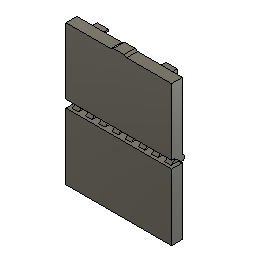
dielectric_frame_box (Autodesk Fusion 360 design; units mm, degrees)
Autodesk Fusion 360 part; units mm, degrees
note: some values were not read from the file. Set by a fixed rule: which face or edge a step refers to.
sketch "Sketch1" plane through (0, 0, 0) normal (0, 0, 1) x (1, 0, 0)
  line L0 (70, 44) -> (-70, 44)
  line L1 (-70, 44) -> (-70, -44)
  line L2 (-70, -44) -> (70, -44)
  line L3 (70, -44) -> (70, 44)
  line L4 (70, 44) -> (-70, -44) construction
  line L5 (-70, 44) -> (70, -44) construction
  dimension "d1" = 140
  dimension "d2" = 88
  constraint horizontal L0
  constraint perpendicular L0 L1
  constraint parallel L0 L2
  constraint parallel L1 L3
  constraint coincident L4 origin
  constraint coincident L5 origin
  measures "d1" distance of L0.start L0.end
  measures "d2" distance of L0.end L1.end
extrude "Extrude1" add sketch "Sketch1" along normal blind 2.5 makes body 1
sketch "Sketch2" plane through (0, 0, 0) normal (0, 0, -1) x (-1, 0, 0)
  line L0 (-70, 44) -> (-70, -44)
  line L1 (-70, -44) -> (70, -44)
  line L2 (70, -44) -> (70, 44)
  line L3 (70, 44) -> (-70, 44)
  line L4 (68.8, 42.8) -> (-68.8, 42.8)
  line L5 (-68.8, 42.8) -> (-68.8, -42.8)
  line L6 (-68.8, -42.8) -> (68.8, -42.8)
  line L7 (68.8, -42.8) -> (68.8, 42.8)
  dimension "d5" = -1.2
sketch "Sketch3" plane through (0, 0, 0) normal (0, 0, -1) x (1, 0, 0)
  line L0 (38, -38.25) -> (38, -31.25)
  line L1 (39, -30.25) -> (42, -30.25)
  line L2 (43, -29.25) -> (43, -26.25)
  line L3 (44, -25.25) -> (51, -25.25)
  line L4 (51, -25.25) -> (51, -38.25)
  line L5 (51, -38.25) -> (38, -38.25)
  line L6 (38, -38.25) -> (38, -40.25)
  line L7 (0, -61) -> (0, 57.3989) construction
  line L8 (91.3753, 0) -> (-120, 0) construction
  arc A0 (42, -30.25) -> (43, -29.25) centre (42, -29.25) ccw
  arc A1 (39, -30.25) -> (38, -31.25) centre (39, -31.25) ccw
  arc A2 (44, -25.25) -> (43, -26.25) centre (44, -26.25) ccw
  line L9 (53, -40.25) -> (53, -25.25)
  line L10 (-68.8, 42.8) -> (-68.8, -42.8)
  line L11 (51, -25.25) -> (53, -25.25)
  line L12 (70, -44) -> (-70, -44) construction
  line L13 (38, -40.25) -> (53, -40.25)
  line L14 (-38, -38.25) -> (-38, -40.25)
  line L15 (-38, -40.25) -> (-53, -40.25)
  line L16 (-53, -40.25) -> (-53, -25.25)
  line L17 (-51, -25.25) -> (-53, -25.25)
  line L18 (-51, -38.25) -> (-38, -38.25)
  line L19 (-51, -25.25) -> (-51, -38.25)
  line L20 (-38, -38.25) -> (-38, -31.25)
  arc A3 (-38, -31.25) -> (-39, -30.25) centre (-39, -31.25) ccw
  line L21 (-39, -30.25) -> (-42, -30.25)
  arc A4 (-43, -29.25) -> (-42, -30.25) centre (-42, -29.25) ccw
  line L22 (-43, -29.25) -> (-43, -26.25)
  arc A5 (-43, -26.25) -> (-44, -25.25) centre (-44, -26.25) ccw
  line L23 (-44, -25.25) -> (-51, -25.25)
  line L24 (38, 38.25) -> (38, 40.25)
  line L25 (38, 40.25) -> (53, 40.25)
  line L26 (51, 25.25) -> (53, 25.25)
  line L27 (53, 40.25) -> (53, 25.25)
  line L28 (51, 38.25) -> (38, 38.25)
  line L29 (51, 25.25) -> (51, 38.25)
  line L30 (38, 38.25) -> (38, 31.25)
  arc A6 (38, 31.25) -> (39, 30.25) centre (39, 31.25) ccw
  line L31 (39, 30.25) -> (42, 30.25)
  arc A7 (43, 29.25) -> (42, 30.25) centre (42, 29.25) ccw
  line L32 (43, 29.25) -> (43, 26.25)
  arc A8 (43, 26.25) -> (44, 25.25) centre (44, 26.25) ccw
  line L33 (44, 25.25) -> (51, 25.25)
  arc A9 (-39, 30.25) -> (-38, 31.25) centre (-39, 31.25) ccw
  line L34 (-39, 30.25) -> (-42, 30.25)
  arc A10 (-42, 30.25) -> (-43, 29.25) centre (-42, 29.25) ccw
  line L35 (-43, 29.25) -> (-43, 26.25)
  arc A11 (-44, 25.25) -> (-43, 26.25) centre (-44, 26.25) ccw
  line L36 (-44, 25.25) -> (-51, 25.25)
  line L37 (-38, 38.25) -> (-38, 31.25)
  line L38 (-51, 38.25) -> (-38, 38.25)
  line L39 (-51, 25.25) -> (-51, 38.25)
  line L40 (-38, 38.25) -> (-38, 40.25)
  line L41 (-38, 40.25) -> (-53, 40.25)
  line L42 (-51, 25.25) -> (-53, 25.25)
  line L43 (-53, 40.25) -> (-53, 25.25)
  point P0 (38, -30.25)
  point P1 (43, -25.25)
  dimension "d10" = 8
  dimension "d11" = 8
  dimension "d12" = 15
  dimension "d13" = 15
  dimension "d14" = 1
  dimension "d15" = 2
  dimension "d48" = 102
  dimension "d49" = 2
  dimension "d85" = 76.5
  constraint vertical L0
  constraint perpendicular L0 L1
  constraint perpendicular L1 L2
  constraint perpendicular L2 L3
  constraint perpendicular L3 L4
  constraint perpendicular L4 L5
  constraint perpendicular L5 L6
  constraint vertical L7
  constraint horizontal L8
  constraint coincident L7 origin
  constraint coincident origin L8
  constraint tangent L1 A0
  constraint tangent L2 A0
  constraint coincident P0 L0
  constraint coincident P0 L1
  constraint tangent L0 A1
  constraint tangent L1 A1
  constraint equal A0 A1
  constraint coincident P1 L2
  constraint coincident P1 L3
  constraint tangent L2 A2
  constraint tangent L3 A2
  constraint equal A0 A2
  constraint equal L4 L5
  constraint perpendicular L4 L11
  constraint perpendicular L9 L13
  constraint symmetric L0.start L7 L14.start
  constraint symmetric L3.end L7 L17.start
  constraint symmetric L4.end L7 L18.start
  constraint symmetric L6.end L7 L14.end
  constraint symmetric L9.start L7 L15.end
  constraint symmetric L7 L1.end L21.end
  constraint symmetric L7 L2.start A4.start
  constraint symmetric L7 A0 A4
  constraint symmetric L7 L0.end L20.end
  constraint symmetric L7 L1.start A3.end
  constraint symmetric L7 A1 A3
  constraint symmetric L7 L2.end L22.end
  constraint symmetric L7 L3.start A5.end
  constraint symmetric L7 A2 A5
  constraint symmetric L7 L9.end L16.end
  constraint symmetric L0.start L8 L24.start
  constraint symmetric L3.end L8 L26.start
  constraint symmetric L4.end L8 L28.start
  constraint symmetric L6.end L8 L24.end
  constraint symmetric L9.start L8 L25.end
  constraint symmetric L8 L1.end L31.end
  constraint symmetric L8 L2.start A7.start
  constraint symmetric L8 A0 A7
  constraint symmetric L8 L0.end L30.end
  constraint symmetric L8 L1.start A6.end
  constraint symmetric L8 A1 A6
  constraint symmetric L8 L2.end L32.end
  constraint symmetric L8 L3.start A8.end
  constraint symmetric L8 A2 A8
  constraint symmetric L8 L9.end L26.end
  constraint symmetric L8 L14.start L37.start
  constraint symmetric L8 L14.end L40.end
  constraint symmetric L8 L15.end L41.end
  constraint symmetric L8 L16.end L42.end
  constraint symmetric L8 L17.start L36.end
  constraint symmetric L8 L18.start L38.start
  constraint symmetric L8 L20.end A9.end
  constraint symmetric L8 A3.end A9.start
  constraint symmetric L8 A3 A9
  constraint symmetric L8 L21.end L34.end
  constraint symmetric L8 A4.start A10.end
  constraint symmetric L8 A4 A10
  constraint symmetric L8 L22.end L35.end
  constraint symmetric L8 A5.end A11.start
  constraint symmetric L8 A5 A11
  measures "d10" distance of L0.start P0
  measures "d11" distance of P1 L3.end
  measures "d12" distance of L6.end L9.start
  measures "d13" distance of L9.start L9.end
  measures "d14" radius of A0
  measures "d15" distance of L0.start L6.end
  measures "d48" distance of L4 L19
  measures "d49" distance of L3.end L9.end
  measures "d85" distance of L5 L28
extrude "Extrude2" add sketch "Sketch3" along normal blind 4 contours L0 L1 L2 L3 L4 L5 A0 A1 A2 | L18 L19 L20 A3 L21 A4 L22 A5 L23 | L28 L29 L30 A6 L31 A7 L32 A8 L33 | A9 L34 A10 L35 A11 L36 L37 L38 L39 bodies 1
extrude "Extrude3" add sketch "Sketch2" along normal blind 12 bodies 1
extrude "Extrude4" add sketch "Sketch3" along normal blind 22 contours L4 L5 L6 L9 L11 L13 | L14 L15 L16 L17 L18 L19 | L24 L25 L26 L27 L28 L29 | L38 L39 L40 L41 L42 L43 bodies 1
ref_plane "WorkPlane1" through (70, 0, -4.75) normal (-1, 0, 0) x (0, -1, 0)
sketch "Sketch4" plane through (70, 0, -10.75) normal (-1, 0, 0) x (0, -1, 0)
  line L0 (44, -1.25) -> (44, 13.25)
  arc A0 (47.2, -3.65) -> (51.2981, 0.6784) centre (49, -1.25) ccw
  circle A1 centre (49, -1.25) radius 1
  line L1 (44, -1.25) -> (47.2, -3.65)
  line L2 (51.2981, 0.6784) -> (44, 9.3759)
  line L3 (44, -1.25) -> (49, -1.25) construction
  dimension "d24" = 3
  dimension "d25" = 2
  dimension "d53" = 5
  dimension "d55" = 140
  constraint concentric A0 A1
  constraint coincident L0.start L1.start
  constraint coincident L0 L2.end
  constraint tangent A0 L2
  constraint tangent A0 L1
  constraint coincident A0.centre A1.centre
  constraint horizontal L3
  measures "d24" radius of A0
  measures "d25" diameter of A1
  measures "d53" horizontal distance of L0.start A0.centre
  measures "d55" angle of L0 L2
extrude "Extrude5" add sketch "Sketch4" along normal mid plane 8.75 separate body makes body 2
pattern_linear "R-Pattern1" count 9 spacing 17.5 along (-1, 0, 0) of bodies 2 makes body 3 at (53.9583, -48.8654, -7.1724) makes body 4 at (36.4583, -48.8654, -7.1724) makes body 5 at (18.9583, -48.8654, -7.1724) makes body 6 at (1.4583, -48.8654, -7.1724) makes body 7 at (-16.0417, -48.8654, -7.1724) makes body 8 at (-33.5417, -48.8654, -7.1724) makes body 9 at (-51.0417, -48.8654, -7.1724) makes body 10 at (-68.5417, -48.8654, -7.1724)
ref_plane "WorkPlane1" through (0, 0, -24) normal (0, 0, -1) x (-1, 0, 0) in component "lid"
sketch "Flat top" plane through (0, 0, -24) normal (0, 0, -1) x (1, 0, 0) in component "lid"
  line L0 (68.8, -42.8) -> (-68.8, -42.8) construction
  line L1 (-68.8, -42.8) -> (-68.8, 42.8) construction
  line L2 (-68.8, 42.8) -> (68.8, 42.8) construction
  line L3 (68.8, 42.8) -> (68.8, -42.8) construction
  line L4 (-70, 44) -> (-70, -44)
  line L5 (-70, -44) -> (70, -44)
  line L6 (70, -44) -> (70, 44)
  line L7 (70, 44) -> (-70, 44)
  line L8 (69.8, -41.8) -> (-69.8, -41.8)
  line L9 (-69.8, -41.8) -> (-69.8, 41.8)
  line L10 (-69.8, 41.8) -> (69.8, 41.8)
  line L11 (69.8, 41.8) -> (69.8, -41.8)
  line L12 (84, 0) -> (65, 0) construction
  constraint horizontal L12
  constraint coincident origin L12
  constraint parallel L0 L8
  constraint parallel L1 L9
  constraint parallel L2 L10
  constraint parallel L3 L11
extrude "Extrude1'" add sketch "Flat top" along normal blind 2.5 separate body contours L4 L5 L6 L7 | L8 L9 L10 L11 makes body 11 in component "lid"
ref_plane "WorkPlane2" through (61.25, -48.5086, -8.6894) normal (1, 0, 0) x (0, 1, 0) in component "lid"
combine "Combine1" operation add target body 1 tool bodies 8 6 3 2 4 5 7 9 10
copy_body "Body->Comp1" bodies 1 removing the originals makes body 12 in component "Component"
ref_plane "WorkPlane3" through (0, 0, -24) normal (0, 0, 1) x (-1, 0, 0) in component "lid"
sketch "Walls" plane through (0, 0, -24) normal (0, 0, 1) x (1, 0, 0) in component "lid"
  line L0 (-68.8, 42.8) -> (-68.8, -42.8)
  line L1 (-68.8, -42.8) -> (68.8, -42.8)
  line L2 (68.8, -42.8) -> (68.8, 42.8)
  line L3 (68.8, 42.8) -> (-68.8, 42.8)
  line L4 (-70, 44) -> (70, 44)
  line L5 (70, 44) -> (70, -44)
  line L6 (70, -44) -> (65.625, -44)
  line L7 (65.625, -44) -> (56.875, -44)
  line L8 (56.875, -44) -> (48.125, -44)
  line L9 (48.125, -44) -> (39.375, -44)
  line L10 (39.375, -44) -> (30.625, -44)
  line L11 (30.625, -44) -> (21.875, -44)
  line L12 (21.875, -44) -> (13.125, -44)
  line L13 (13.125, -44) -> (4.375, -44)
  line L14 (4.375, -44) -> (-4.375, -44)
  line L15 (-4.375, -44) -> (-13.125, -44)
  line L16 (-13.125, -44) -> (-21.875, -44)
  line L17 (-21.875, -44) -> (-30.625, -44)
  line L18 (-30.625, -44) -> (-39.375, -44)
  line L19 (-39.375, -44) -> (-48.125, -44)
  line L20 (-48.125, -44) -> (-56.875, -44)
  line L21 (-56.875, -44) -> (-65.625, -44)
  line L22 (-65.625, -44) -> (-70, -44)
  line L23 (-70, -44) -> (-70, 44)
extrude "Extrude4'" add sketch "Walls" along normal blind 12 separate body makes body 13 in component "lid"
sketch "Hinge profile" plane through (61.25, -46.2271, -22.2758) normal (1, 0, 0) x (0, 0, -1) in component "lid"
  line L0 (1.7242, 2.2271) -> (4.2242, 2.2271)
  circle A0 centre (-10.2758, -2.7729) radius 1.5
  arc A1 (-12.6758, -0.9729) -> (-8.3474, -5.071) centre (-10.2758, -2.7729) ccw
  line L1 (4.2242, 90.2271) -> (4.2242, 2.2271)
  line L2 (1.7242, 2.2271) -> (-10.2758, 2.2271)
  line L3 (-12.6758, -0.9729) -> (-10.2758, 2.2271)
  line L4 (-8.3474, -5.071) -> (0.3502, 2.2271)
  line L5 (-10.2758, -2.7729) -> (-10.2758, 2.2271) construction
  dimension "d59" = 3
  dimension "d60" = 1.5
  dimension "d64" = 5
  dimension "d65" = 12
  dimension "d89" = 140
  constraint coincident A0.centre A1.centre
  constraint coincident L2.end L3.end
  constraint coincident L2 L4.end
  constraint vertical L5
  constraint tangent A1 L4
  constraint tangent A1 L3
  measures "d59" diameter of A0
  measures "d60" distance of A0 A1
  measures "d64" distance of L0 A0.centre
  measures "d65" horizontal distance of L0.start A0.centre
  measures "d89" angle of L2 L4
extrude "Extrude2'" add sketch "Hinge profile" along normal mid plane 8.25 separate body makes body 14 in component "lid"
sketch "Sketch3 (2)" plane through (0, 0, -24) normal (0, 0, 1) x (1, 0, 0) in component "lid"
  line L0 (-69.3, 40.8) -> (69.3, 40.8)
  line L1 (69.3, 40.8) -> (69.3, -41.05)
  line L2 (69.3, -41.05) -> (-69.3, -41.05)
  line L3 (-69.3, -41.05) -> (-69.3, 40.8)
  line L4 (-67.8, 39.3) -> (67.8, 39.3)
  line L5 (67.8, 39.3) -> (67.8, -39.55)
  line L6 (67.8, -39.55) -> (-67.8, -39.55)
  line L7 (-67.8, -39.55) -> (-67.8, 39.3)
  line L8 (69.8, 41.8) -> (-69.8, 41.8)
  line L9 (69.8, -41.8) -> (69.8, 41.8)
  line L10 (-69.8, -41.8) -> (69.8, -41.8)
  line L11 (-69.8, 41.8) -> (-69.8, -41.8)
  line L12 (-70, -44) -> (70, -44)
  line L13 (70, -44) -> (70, 44)
  line L14 (70, 44) -> (-70, 44)
  line L15 (-70, 44) -> (-70, -44)
  dimension "d72" = 1
  dimension "d73" = 0.5
  dimension "d75" = 0.75
  dimension "d76" = 0.5
  dimension "d77" = 1.5
  dimension "d78" = 1.5
  dimension "d79" = 1.5
  dimension "d80" = 1.5
  constraint horizontal L0
  constraint vertical L1
  constraint horizontal L2
  constraint vertical L3
  constraint horizontal L4
  constraint vertical L5
  constraint horizontal L6
  constraint vertical L7
  measures "d72" distance of L0 L8
  measures "d73" distance of L1 L9
  measures "d75" distance of L2 L10
  measures "d76" distance of L3 L11
  measures "d77" distance of L3 L7
  measures "d78" distance of L2 L6
  measures "d79" distance of L1 L5
  measures "d80" distance of L0 L4
sketch "latch extrude" plane through (0, -97.9819, -24) normal (0, 0, 1) x (-1, 0, 0) in component "lid"
  line L0 (70, -53.9819) -> (-70, -53.9819)
  line L1 (-70, -53.9819) -> (-70, -141.9819)
  line L2 (-70, -141.9819) -> (70, -141.9819)
  line L3 (70, -141.9819) -> (70, -53.9819)
  line L4 (-5, -138.9819) -> (-5, -141.9819)
  line L5 (-5, -141.9819) -> (5, -141.9819)
  line L6 (5, -141.9819) -> (5, -138.9819)
  line L7 (5, -138.9819) -> (-5, -138.9819)
  line L8 (0, 80) -> (0, -240) construction
  line L9 (68.8, -140.7819) -> (-68.8, -140.7819)
  point P0 (0, -138.9819)
  dimension "d90" = 10
  dimension "d91" = 3
  constraint perpendicular L2 L4
  constraint perpendicular L4 L5
  constraint perpendicular L2 L6
  constraint perpendicular L4 L7
  constraint coincident L2 L4.end
  constraint vertical L8
  constraint midpoint L7 P0
  constraint coincident L8 P0
  constraint coincident origin L8
  measures "d90" distance of L4.start L6.end
  measures "d91" distance of L5.end L6.end
extrude "Extrude5'" add sketch "latch extrude" along normal blind 18 contours L4 L6 L7 L9 bodies 13 11 in component "lid"
sketch "Sketch6 (1)" plane through (-5, 0, 0) normal (-1, 0, 0) x (0, 0, 1) in component "lid"
  line L0 (-12, 42.8) -> (-24, 42.8)
  line L1 (-24, 42.8) -> (-24, 41)
  line L2 (-24, 41) -> (-6, 41)
  line L3 (-6, 41) -> (-6, 42.8)
  line L4 (-9, 42.8) -> (-8.0668, 43.583)
  line L5 (-7.7454, 43.7) -> (-7.2546, 43.7)
  line L6 (-6.9332, 43.583) -> (-6, 42.8)
  arc A0 (-6.9332, 43.583) -> (-7.2546, 43.7) centre (-7.2546, 43.2) ccw
  arc A1 (-7.7454, 43.7) -> (-8.0668, 43.583) centre (-7.7454, 43.2) ccw
  line L7 (-6, 42.8) -> (-12, 42.8)
  dimension "d95" = 3
  dimension "d96" = 140
  dimension "d97" = 0.5
  dimension "d98" = 0.5
  dimension "d118" = 140
  dimension "d119" = 0.9
  constraint tangent L5 A0
  constraint tangent L6 A0
  constraint tangent L4 A1
  constraint tangent L5 A1
  constraint coincident L4.start L7
  constraint coincident L3.end L6.end
  measures "d95" distance of L4.start L3.end
  measures "d96" angle of L5 L6
  measures "d97" radius of A0
  measures "d98" radius of A1
  measures "d118" angle of L4 L5
  measures "d119" distance of L5 L7
extrude "Extrude6" add sketch "Sketch6 (1)" against normal up to surface (10 mm away) contours L4 L5 L6 A0 A1 L7 bodies 13 in component "lid"
sketch "Sketch1 (2)" plane through (0, 42.8, 0) normal (0, -1, 0) x (1, 0, 0) in component "Component"
  line L0 (68.8, 0) -> (-68.8, 0)
  line L1 (-68.8, 0) -> (-68.8, -12)
  line L2 (-68.8, -12) -> (68.8, -12)
  line L3 (68.8, -12) -> (68.8, 0)
  line L4 (0, -22) -> (0, 3) construction
  line L5 (6, -4) -> (-6, -4)
  line L6 (-6, -4) -> (-6, -12)
  line L7 (-6, -12) -> (6, -12)
  line L8 (6, -12) -> (6, -4)
  point P0 (0, -12)
  point P1 (0, -4)
  dimension "d102" = 12
  dimension "d103" = 8
  constraint perpendicular L2 L4
  constraint midpoint L2 P0
  constraint coincident L4 P0
  constraint horizontal L5
  constraint vertical L6
  constraint horizontal L7
  constraint vertical L8
  constraint coincident L2 L6.end
  constraint midpoint L5 P1
  constraint coincident L4 P1
  measures "d102" distance of L5.start L5.end
  measures "d103" distance of L5.end L6.end
extrude "Extrude1''" cut sketch "Sketch1 (2)" against normal blind 1.3 contours L2 L5 L6 L7 L8 bodies 12 in component "Component"
sketch "Sketch2 (2)" plane through (0, 0, 2.5) normal (0, 0, 1) x (1, 0, 0) in component "Component"
  line L0 (70, -44) -> (70, 44)
  line L1 (70, 44) -> (-70, 44)
  line L2 (-70, 44) -> (-70, -44)
  line L3 (-70, -44) -> (70, -44)
  line L4 (-10.4641, 44) -> (-7, 46)
  line L5 (-7, 46) -> (7, 46)
  line L6 (7, 46) -> (10.4641, 44)
  line L7 (0, 57) -> (0, 37) construction
  point P0 (0, 46)
  dimension "d107" = 150
  dimension "d108" = 14
  dimension "d109" = 2
  constraint coincident L1 L4.start
  constraint parallel L1 L5
  constraint coincident L1 L6.end
  constraint vertical L7
  constraint coincident origin L7
  constraint midpoint L5 P0
  constraint coincident L7 P0
  constraint symmetric L4 L6 L7
  measures "d107" angle of L4 L5
  measures "d108" distance of L4.end L5.end
  measures "d109" distance of L1 L5
extrude "Extrude2''" add sketch "Sketch2 (2)" against normal up to surface (14.5 mm away) contours L1 L4 L5 L6 bodies 12 in component "Component"
sketch "Sketch3 (3)" plane through (6, 0, 0) normal (-1, 0, 0) x (0, 0, 1) in component "Component"
  line L0 (-4, 44) -> (-12, 44)
  line L1 (-12, 44) -> (-12, 42.8)
  line L2 (-12, 42.8) -> (-4, 42.8)
  line L3 (-4, 42.8) -> (-4, 44)
  line L4 (-10.7679, 44) -> (-9.8347, 43.217)
  line L5 (-9.5133, 43.1) -> (-9.0867, 43.1)
  line L6 (-8.7653, 43.217) -> (-7.8321, 44)
  arc A0 (-9.8347, 43.217) -> (-9.5133, 43.1) centre (-9.5133, 43.6) ccw
  arc A1 (-9.0867, 43.1) -> (-8.7653, 43.217) centre (-9.0867, 43.6) ccw
  point P0 (-9.3, 43.1)
  dimension "d112" = 0.5
  dimension "d113" = 0.9
  dimension "d114" = 2.7
  dimension "d120" = 140
  dimension "d122" = 140
  constraint coincident L0 L4.start
  constraint parallel L0 L5
  constraint coincident L0 L6.end
  constraint tangent L4 A0
  constraint tangent L5 A0
  constraint tangent L5 A1
  constraint tangent L6 A1
  constraint equal A0 A1
  constraint midpoint L5 P0
  measures "d112" radius of A0
  measures "d113" distance of L0 L5
  measures "d114" distance of L1 P0
  measures "d120" angle of L4 L5
  measures "d122" angle of L5 L6
extrude "Extrude3'" add sketch "Sketch3 (3)" along normal up to surface (12 mm away) contours L0 L4 L5 L6 A0 A1 bodies 12 in component "Component"
pattern_linear "R-Pattern1'" count 8 spacing 17.5 along (-1, 0, 0) of bodies 14 makes body 15 at (45.125, -48.8654, -16.8276) makes body 16 at (27.625, -48.8654, -16.8276) makes body 17 at (10.125, -48.8654, -16.8276) makes body 18 at (-7.375, -48.8654, -16.8276) makes body 19 at (-24.875, -48.8654, -16.8276) makes body 20 at (-42.375, -48.8654, -16.8276) makes body 21 at (-59.875, -48.8654, -16.8276) in component "lid"
extrude "Extrude4''" cut 1 faces at (74.375, -45.4588, -8.1974) along direction (-1, 0, 0) up to surface (4.375 mm away) on bodies 12 bodies 12 in component "Component"
extrude "Extrude5''" cut 1 faces at (-74.375, -45.4588, -8.1974) along direction (1, 0, 0) up to surface (4.375 mm away) on bodies 12 bodies 12 in component "Component"
sketch "Sketch7" plane through (-70, 0, 0) normal (-1, 0, 0) x (0, 0, 1)
  circle A0 centre (-12, -49) radius 1
  line L0 (-1.3741, -44) -> (2.5, -44)
  line L1 (2.5, -44) -> (2.5, 44)
  line L2 (2.5, 44) -> (-12, 44)
  line L3 (-12, 44) -> (-12, -44)
  line L4 (-12, -44) -> (-14.4, -47.2)
  arc A1 (-14.4, -47.2) -> (-10.0716, -51.2981) centre (-12, -49) ccw
  line L5 (-10.0716, -51.2981) -> (-1.3741, -44)
extrude "Extrude6'" add sketch "Sketch7" against normal up to surface (140 mm away) contours A0 bodies 12 in component "Component"
sketch "Sketch7 (2)" plane through (0, 0, -24) normal (0, 0, 1) x (1, 0, 0) in component "lid"
  line L0 (-5, 41) -> (-5, 42.8)
  line L1 (-5, 42.8) -> (-68.8, 42.8)
  line L2 (-68.8, 42.8) -> (-68.8, -42.8)
  line L3 (-68.8, -42.8) -> (68.8, -42.8)
  line L4 (68.8, -42.8) -> (68.8, 42.8)
  line L5 (68.8, 42.8) -> (5, 42.8)
  line L6 (5, 42.8) -> (5, 41)
  line L7 (5, 41) -> (-5, 41)
  arc A0 (-43, -26.25) -> (-44, -25.25) centre (-44, -26.25) ccw construction
  line L8 (-43, -26.25) -> (-43, -29.25) construction
  arc A1 (-43, -29.25) -> (-42, -30.25) centre (-42, -29.25) ccw construction
  line L9 (-42, -30.25) -> (-39, -30.25) construction
  arc A2 (-38, -31.25) -> (-39, -30.25) centre (-39, -31.25) ccw construction
  line L10 (-38, -31.25) -> (-38, -38.25) construction
  line L11 (-38, -38.25) -> (-51, -38.25) construction
  line L12 (-51, -38.25) -> (-51, -25.25) construction
  line L13 (-51, -25.25) -> (-44, -25.25) construction
  line L14 (43, -29.25) -> (43, -26.25) construction
  arc A3 (44, -25.25) -> (43, -26.25) centre (44, -26.25) ccw construction
  line L15 (44, -25.25) -> (51, -25.25) construction
  line L16 (51, -25.25) -> (51, -38.25) construction
  line L17 (51, -38.25) -> (38, -38.25) construction
  line L18 (38, -38.25) -> (38, -31.25) construction
  arc A4 (39, -30.25) -> (38, -31.25) centre (39, -31.25) ccw construction
  line L19 (39, -30.25) -> (42, -30.25) construction
  arc A5 (42, -30.25) -> (43, -29.25) centre (42, -29.25) ccw construction
  line L20 (51, 25.25) -> (44, 25.25) construction
  arc A6 (43, 26.25) -> (44, 25.25) centre (44, 26.25) ccw construction
  line L21 (43, 26.25) -> (43, 29.25) construction
  arc A7 (43, 29.25) -> (42, 30.25) centre (42, 29.25) ccw construction
  line L22 (42, 30.25) -> (39, 30.25) construction
  arc A8 (38, 31.25) -> (39, 30.25) centre (39, 31.25) ccw construction
  line L23 (38, 31.25) -> (38, 38.25) construction
  line L24 (38, 38.25) -> (51, 38.25) construction
  line L25 (51, 38.25) -> (51, 25.25) construction
  line L26 (-43, 29.25) -> (-43, 26.25) construction
  arc A9 (-44, 25.25) -> (-43, 26.25) centre (-44, 26.25) ccw construction
  line L27 (-44, 25.25) -> (-51, 25.25) construction
  line L28 (-51, 25.25) -> (-51, 38.25) construction
  line L29 (-51, 38.25) -> (-38, 38.25) construction
  line L30 (-38, 38.25) -> (-38, 31.25) construction
  arc A10 (-39, 30.25) -> (-38, 31.25) centre (-39, 31.25) ccw construction
  line L31 (-39, 30.25) -> (-42, 30.25) construction
  arc A11 (-42, 30.25) -> (-43, 29.25) centre (-42, 29.25) ccw construction
  line L32 (-49.5, -26.75) -> (-44.5, -26.75)
  line L33 (-49.5, -36.75) -> (-49.5, -26.75)
  line L34 (-39.5, -36.75) -> (-49.5, -36.75)
  line L35 (-39.5, -31.75) -> (-39.5, -36.75)
  line L36 (-42, -31.75) -> (-39.5, -31.75)
  arc A12 (-44.5, -29.25) -> (-42, -31.75) centre (-42, -29.25) ccw
  line L37 (-44.5, -26.75) -> (-44.5, -29.25)
  line L38 (39.5, -36.75) -> (39.5, -31.75)
  line L39 (39.5, -31.75) -> (42, -31.75)
  arc A13 (42, -31.75) -> (44.5, -29.25) centre (42, -29.25) ccw
  line L40 (44.5, -29.25) -> (44.5, -26.75)
  line L41 (44.5, -26.75) -> (49.5, -26.75)
  line L42 (49.5, -26.75) -> (49.5, -36.75)
  line L43 (49.5, -36.75) -> (39.5, -36.75)
  line L44 (-39.5, 36.75) -> (-39.5, 31.75)
  line L45 (-49.5, 36.75) -> (-39.5, 36.75)
  line L46 (-49.5, 26.75) -> (-49.5, 36.75)
  line L47 (-44.5, 26.75) -> (-49.5, 26.75)
  line L48 (-44.5, 29.25) -> (-44.5, 26.75)
  arc A14 (-42, 31.75) -> (-44.5, 29.25) centre (-42, 29.25) ccw
  line L49 (-39.5, 31.75) -> (-42, 31.75)
  line L50 (49.5, 26.75) -> (44.5, 26.75)
  line L51 (44.5, 26.75) -> (44.5, 29.25)
  arc A15 (44.5, 29.25) -> (42, 31.75) centre (42, 29.25) ccw
  line L52 (42, 31.75) -> (39.5, 31.75)
  line L53 (39.5, 31.75) -> (39.5, 36.75)
  line L54 (39.5, 36.75) -> (49.5, 36.75)
  line L55 (49.5, 36.75) -> (49.5, 26.75)
  dimension "d135" = 1.5
  dimension "d136" = 1.5
  dimension "d137" = 1.5
  dimension "d138" = 1.5
extrude "Extrude7" add sketch "Sketch7 (2)" along normal up to surface (2.25 mm away) contours L32 L33 L34 L35 L36 A12 L37 | L38 L39 A13 L40 L41 L42 L43 | L44 L45 L46 L47 L48 A14 L49 | L50 L51 A15 L52 L53 L54 L55 bodies 13 in component "lid"
sketch "inner seal" plane through (0, 0, -12) normal (0, 0, 1) x (1, 0, 0) in component "lid"
  line L0 (-68.8, 42.8) -> (-5, 42.8)
  line L1 (-5, 42.8) -> (5, 42.8)
  line L2 (5, 42.8) -> (68.8, 42.8)
  line L3 (68.8, 42.8) -> (68.8, -42.8)
  line L4 (68.8, -42.8) -> (-68.8, -42.8)
  line L5 (-68.8, -42.8) -> (-68.8, 42.8)
  line L6 (-70, -44) -> (70, -44)
  line L7 (70, -44) -> (70, 44)
  line L8 (70, 44) -> (-70, 44)
  line L9 (-70, 44) -> (-70, -44)
  line L10 (67.8, 41.8) -> (67.8, -41.8)
  line L11 (-67.8, -41.8) -> (-67.8, 41.8)
  line L12 (66.3, 40.3) -> (66.3, -40.3)
  line L13 (-66.3, -40.3) -> (-66.3, 40.3)
  line L14 (-6, 40.3) -> (-6, 41.8)
  line L15 (6, 40.3) -> (6, 41.8)
  line L16 (0, 16) -> (0, -15) construction
  line L17 (38, 40.25) -> (53, 40.25)
  line L18 (-53, 40.25) -> (-38, 40.25)
  line L19 (-37.25, 40.3) -> (-37.25, 41.8)
  line L20 (-53.75, 40.3) -> (-53.75, 41.8)
  line L21 (37.25, 40.3) -> (37.25, 41.8)
  line L22 (53.75, 40.3) -> (53.75, 41.8)
  line L23 (6, 40.3) -> (37.25, 40.3)
  line L24 (53.75, 40.3) -> (66.3, 40.3)
  line L25 (-66.3, 40.3) -> (-53.75, 40.3)
  line L26 (-37.25, 40.3) -> (-6, 40.3)
  line L27 (53.75, -40.3) -> (53.75, -41.8)
  line L28 (37.25, -40.3) -> (37.25, -41.8)
  line L29 (-37.25, -40.3) -> (-37.25, -41.8)
  line L30 (-53.75, -40.3) -> (-53.75, -41.8)
  line L31 (-53.75, -40.3) -> (-66.3, -40.3)
  line L32 (66.3, -40.3) -> (53.75, -40.3)
  line L33 (37.25, -40.3) -> (-37.25, -40.3)
  line L34 (-53.75, 41.8) -> (-53.75, 42.8)
  line L35 (-37.25, 41.8) -> (-37.25, 42.8)
  line L36 (-67.8, 41.8) -> (-53.75, 41.8)
  line L37 (6, 41.8) -> (6, 42.8)
  line L38 (-6, 41.8) -> (-6, 42.8)
  line L39 (-37.25, 41.8) -> (-6, 41.8)
  line L40 (37.25, 41.8) -> (37.25, 42.8)
  line L41 (53.75, 41.8) -> (53.75, 42.8)
  line L42 (6, 41.8) -> (37.25, 41.8)
  line L43 (53.75, 41.8) -> (67.8, 41.8)
  line L44 (53.75, -41.8) -> (53.75, -42.8)
  line L45 (37.25, -41.8) -> (37.25, -42.8)
  line L46 (67.8, -41.8) -> (53.75, -41.8)
  line L47 (-53.75, -41.8) -> (-53.75, -42.8)
  line L48 (-37.25, -41.8) -> (-37.25, -42.8)
  line L49 (37.25, -41.8) -> (-37.25, -41.8)
  line L50 (-53.75, -41.8) -> (-67.8, -41.8)
  dimension "d141" = 1.5
  dimension "d142" = 1.5
  dimension "d143" = 1.5
  dimension "d144" = 1.5
  dimension "d145" = 1
  dimension "d146" = 1
  dimension "d147" = 1
  dimension "d148" = 1
  dimension "d149" = 12
  dimension "d162" = 0.75
  dimension "d163" = 0.75
  dimension "d164" = 0.75
  dimension "d165" = 0.75
  dimension "d166" = 0.75
  dimension "d167" = 0.75
  dimension "d168" = 0.75
  dimension "d169" = 0.75
  constraint horizontal L36
  constraint vertical L10
  constraint horizontal L46
  constraint vertical L11
  constraint horizontal L25
  constraint vertical L12
  constraint horizontal L32
  constraint vertical L13
  constraint coincident L14.end L36
  constraint perpendicular L14 L36
  constraint coincident L15.start L25
  constraint coincident L15.end L36
  constraint perpendicular L15 L36
  constraint collinear L23 L25
  constraint vertical L16
  constraint coincident origin L16
  constraint symmetric L14 L15 L16
  constraint coincident L19.start L25
  constraint coincident L19.end L36
  constraint perpendicular L19 L36
  constraint perpendicular L20 L36
  constraint coincident L21.end L36
  constraint perpendicular L21 L36
  constraint coincident L22.start L23
  constraint coincident L22.end L36
  constraint perpendicular L22 L36
  constraint collinear L23 L24
  constraint collinear L25 L26
  constraint perpendicular L27 L46
  constraint coincident L28.start L32
  constraint coincident L28.end L46
  constraint perpendicular L28 L46
  constraint coincident L29.end L46
  constraint perpendicular L29 L46
  constraint coincident L30.start L32
  constraint coincident L30.end L46
  constraint perpendicular L30 L46
  constraint collinear L31 L32
  constraint collinear L32 L33
  constraint coincident L0 L34.end
  constraint perpendicular L0 L34
  constraint coincident L0 L35.end
  constraint perpendicular L0 L35
  constraint collinear L36 L39
  constraint coincident L2 L37.end
  constraint perpendicular L2 L37
  constraint coincident L0 L38.end
  constraint perpendicular L0 L38
  constraint collinear L39 L42
  constraint coincident L2 L40.end
  constraint perpendicular L2 L40
  constraint coincident L2 L41.end
  constraint perpendicular L2 L41
  constraint collinear L42 L43
  constraint coincident L4 L44.end
  constraint perpendicular L4 L44
  constraint coincident L4 L45.end
  constraint perpendicular L4 L45
  constraint collinear L46 L49
  constraint coincident L4 L47.end
  constraint perpendicular L4 L47
  constraint coincident L4 L48.end
  constraint perpendicular L4 L48
  constraint collinear L49 L50
  measures "d141" distance of L25 L36
  measures "d142" distance of L11 L13
  measures "d143" distance of L32 L46
  measures "d144" distance of L10 L12
  measures "d145" distance of L0 L36
  measures "d146" distance of L5 L11
  measures "d147" distance of L3 L10
  measures "d148" distance of L4 L46
  measures "d149" distance of L14 L15
  measures "d162" distance of L18.end L19
  measures "d163" distance of L18.start L20
  measures "d164" distance of L17.start L21
  measures "d165" distance of L17.end L22
  measures "d166" distance of L17.end L27
  measures "d167" distance of L17.start L28
  measures "d168" distance of L18.end L29
  measures "d169" distance of L18.start L30
extrude "Extrude8" add sketch "inner seal" against normal blind 3 contours L0 L4 L5 L11 L34 L36 L47 L50 | L0 L35 L38 L39 | L11 L13 L20 L25 L30 L31 L36 L50 | L14 L19 L26 L39 | L4 L45 L48 L49 | L28 L29 L33 L49 | L2 L3 L4 L10 L41 L43 L44 L46 | L2 L37 L40 L42 | L10 L12 L22 L24 L27 L32 L43 L46 | L15 L21 L23 L42 bodies 13 in component "lid"
extrude "Extrude9" add sketch "inner seal" along normal blind 1.5 contours L11 L13 L20 L25 L30 L31 L36 L50 | L14 L19 L26 L39 | L28 L29 L33 L49 | L10 L12 L22 L24 L27 L32 L43 L46 | L15 L21 L23 L42 bodies 13 in component "lid"
chamfer "Chamfer1" distance 3 distance2 2.5 6 edges at (61.275, 42.8, -15) (-61.275, 42.8, -15) (21.625, 42.8, -15) (-21.625, 42.8, -15) (68.8, 0, -15) (-68.8, 0, -15) measured on face at (37.0167, 42.8, -21) measured on face at (-37.0167, 42.8, -21) measured on face at (37.0167, 42.8, -21) measured on face at (-37.0167, 42.8, -21) measured on face at (68.8, 14.2667, -18) measured on face at (-68.8, 14.2667, -21) on bodies 13 in component "lid"
chamfer "Chamfer2" distance 3 distance2 2.5 3 edges at (60.025, -42.8, -15) (-60.025, -42.8, -15) (0, -42.8, -15) measured on face at (-12.4167, -42.8, -21) measured on face at (-12.4167, -42.8, -21) measured on face at (-12.4167, -42.8, -21) on bodies 13 in component "lid"
sketch "Sketch9" plane through (0, 0, -12) normal (0, 0, 1) x (1, 0, 0) in component "lid"
  line L0 (-5, 42.8) -> (5, 42.8)
  line L1 (-70, -44) -> (70, -44)
  line L2 (70, -44) -> (70, 44)
  line L3 (70, 44) -> (-70, 44)
  line L4 (-70, 44) -> (-70, -44)
  line L5 (-67.8, -41.8) -> (67.8, -41.8)
  line L6 (67.8, -41.8) -> (67.8, -44)
  line L7 (67.8, -44) -> (-67.8, -44)
  line L8 (-67.8, -44) -> (-67.8, -41.8)
  line L9 (37.25, -41.8) -> (-37.25, -41.8)
  line L10 (-37.25, -41.8) -> (-37.25, -42.8)
  line L11 (-37.25, -42.8) -> (-53.75, -42.8)
  line L12 (-53.75, -42.8) -> (-53.75, -41.8)
  line L13 (-53.75, -41.8) -> (-67.8, -41.8)
  line L14 (-67.8, -41.8) -> (-67.8, 41.8)
  line L15 (-67.8, 41.8) -> (-53.75, 41.8)
  line L16 (-53.75, 41.8) -> (-53.75, 42.8)
  line L17 (-53.75, 42.8) -> (-37.25, 42.8)
  line L18 (-37.25, 42.8) -> (-37.25, 41.8)
  line L19 (-37.25, 41.8) -> (-6, 41.8)
  line L20 (-6, 41.8) -> (-6, 42.8)
  line L21 (-6, 42.8) -> (-5, 42.8)
  line L22 (5, 42.8) -> (6, 42.8)
  line L23 (6, 42.8) -> (6, 41.8)
  line L24 (6, 41.8) -> (37.25, 41.8)
  line L25 (37.25, 41.8) -> (37.25, 42.8)
  line L26 (37.25, 42.8) -> (53.75, 42.8)
  line L27 (53.75, 42.8) -> (53.75, 41.8)
  line L28 (53.75, 41.8) -> (67.8, 41.8)
  line L29 (67.8, 41.8) -> (67.8, -41.8)
  line L30 (67.8, -41.8) -> (53.75, -41.8)
  line L31 (53.75, -41.8) -> (53.75, -42.8)
  line L32 (53.75, -42.8) -> (37.25, -42.8)
  line L33 (37.25, -42.8) -> (37.25, -41.8)
  point P0 (67.8, -41.8)
  constraint horizontal L5
  constraint vertical L6
  constraint horizontal L7
  constraint vertical L8
  constraint coincident L1 L6.end
  constraint coincident P0 L5.end
extrude "Extrude10" cut sketch "Sketch9" against normal blind 0.2 contours L1 L5 L6 L7 L8 L9 L10 L11 L12 L13 L30 L31 L32 L33 | L5 L10 L11 L12 | L5 L31 L32 L33 bodies 13 in component "lid"
sketch "Sketch4 (2)" plane through (0, 0, -12) normal (0, 0, -1) x (-1, 0, 0) in component "Component"
  line L0 (6, 44) -> (6, 42.8)
  line L1 (6, 42.8) -> (68.8, 42.8)
  line L2 (68.8, 42.8) -> (68.8, -42.8)
  line L3 (68.8, -42.8) -> (-68.8, -42.8)
  line L4 (-68.8, -42.8) -> (-68.8, 42.8)
  line L5 (-68.8, 42.8) -> (-6, 42.8)
  line L6 (-6, 42.8) -> (-6, 44)
  line L7 (-6, 44) -> (6, 44)
  line L8 (10.4641, 44) -> (7, 46)
  line L9 (7, 46) -> (-7, 46)
  line L10 (-7, 46) -> (-10.4641, 44)
  line L11 (-10.4641, 44) -> (-70, 44)
  line L12 (-70, 44) -> (-70, -44)
  line L13 (-70, -44) -> (-65.625, -44)
  line L14 (-65.625, -44) -> (-56.875, -44)
  line L15 (-56.875, -44) -> (-48.125, -44)
  line L16 (-48.125, -44) -> (-39.375, -44)
  line L17 (-39.375, -44) -> (-30.625, -44)
  line L18 (-30.625, -44) -> (-21.875, -44)
  line L19 (-21.875, -44) -> (-13.125, -44)
  line L20 (-13.125, -44) -> (-4.375, -44)
  line L21 (-4.375, -44) -> (4.375, -44)
  line L22 (4.375, -44) -> (13.125, -44)
  line L23 (13.125, -44) -> (21.875, -44)
  line L24 (21.875, -44) -> (30.625, -44)
  line L25 (30.625, -44) -> (39.375, -44)
  line L26 (39.375, -44) -> (48.125, -44)
  line L27 (48.125, -44) -> (56.875, -44)
  line L28 (56.875, -44) -> (65.625, -44)
  line L29 (65.625, -44) -> (70, -44)
  line L30 (70, -44) -> (70, 44)
  line L31 (70, 44) -> (10.4641, 44)
  line L32 (68.8, -42.8) -> (68.8, -44)
  line L33 (-68.8, -42.8) -> (-68.8, -44)
  constraint coincident L2.end L3.start
  constraint coincident L29 L32.end
  constraint perpendicular L29 L32
  constraint coincident L3.end L4.start
  constraint coincident L13 L33.end
  constraint perpendicular L13 L33
extrude "Extrude7'" [suppressed] in component "Component"
component "lid" placed x (1, 0, 0) y (0, 1, 0) z (0, 0, 1) at (0, 0, 0)
component "Component" placed x (1, 0, 0) y (0, 1, 0) z (0, 0, 1) at (0, 0, 0)
equation "hinge_pitch = 8.75 mm"
equation "d30 = -hinge_pitch / 2"
equation "d33 = -hinge_pitch * 2"
equation "d61 = hinge_pitch / 2 - 0.25 mm"
equation "d125 = -hinge_pitch * 2"
